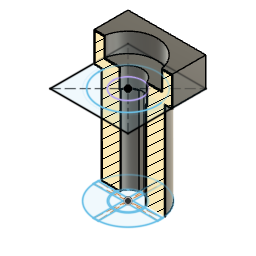
Expansion Anchor v8 (Autodesk Fusion 360 design; units mm, degrees)
Autodesk Fusion 360 part; units mm, degrees
note: some values were not read from the file. Set by a fixed rule: which sketch regions a step uses.
sketch "Schizzo1" plane through (0, 0, 0) normal (0, 0, 1) x (1, 0, 0)
  circle A0 centre (10.2944, 3.2873) radius 1.4
  circle A1 centre (10.2944, 3.2873) radius 3.3
  line L0 (13.5944, 3.0373) -> (6.9944, 3.0373)
  line L1 (6.9944, 3.0373) -> (6.9944, 3.5373)
  line L2 (6.9944, 3.5373) -> (13.5944, 3.5373)
  line L3 (13.5944, 3.5373) -> (13.5944, 3.0373)
  line L4 (13.5944, 3.0373) -> (6.9944, 3.5373) construction
  line L5 (6.9944, 3.0373) -> (13.5944, 3.5373) construction
  line L6 (10.5444, -0.0127) -> (10.0444, -0.0127)
  line L7 (10.0444, -0.0127) -> (10.0444, 6.5873)
  line L8 (10.0444, 6.5873) -> (10.5444, 6.5873)
  line L9 (10.5444, 6.5873) -> (10.5444, -0.0127)
  line L10 (10.5444, -0.0127) -> (10.0444, 6.5873) construction
  line L11 (10.0444, -0.0127) -> (10.5444, 6.5873) construction
  circle A2 centre (10.2944, 3.2873) radius 1.5
  point P0 (10.2944, 3.2873)
  point P1 (10.2944, 3.2873)
  dimension "d1" = 2.8
  dimension "d2" = 6.6
  dimension "d3" = 0.5
  dimension "d4" = 0.5
  dimension "d16" = 3
  constraint concentric A0 A1
  constraint horizontal L0
  constraint perpendicular L0 L1
  constraint parallel L0 L2
  constraint parallel L1 L3
  constraint coincident L4 P1
  constraint coincident L5 P1
  constraint coincident P0 A0.centre
  constraint horizontal L6
  constraint perpendicular L6 L7
  constraint parallel L6 L8
  constraint parallel L7 L9
  constraint coincident L10 P1
  constraint coincident L11 P1
  constraint coincident P1 P0
  constraint tangent A1 L1
  constraint tangent A1 L8
  constraint concentric A1 A2
  measures "d1" diameter of A0
  measures "d2" diameter of A1
  measures "d3" distance of L0.end L1.end
  measures "d4" distance of L7.end L8.end
  measures "d16" diameter of A2
extrude "Estrusione1" add sketch "Schizzo1" along normal blind 9 contours A0 L2 L9 A2 | A0 L0 L9 A2 | A1 L2 L9 A2 | A1 L0 L9 A2 | A0 L2 L7 A2 | A0 L0 L7 A2 | A1 L2 L7 A2 | A1 L0 L7 A2 makes body 1 at (7.1541, 4.3014, 6) makes body 2 at (7.5637, 1.4344, 6) makes body 3 at (12.397, 5.8308, 6) makes body 4 at (13.3249, 1.9811, 6)
extrude "Estrusione2" add sketch "Schizzo1" along normal blind 1 from surface at 9 contours A1 L2 L9 A2 | A1 L0 L2 A2 | A1 L0 L9 A2 | A1 L7 L9 A2 | A1 L7 L9 A2 | A1 L2 L7 A2 | A1 L0 L7 A2 | A1 L0 L2 A2 bodies 1 2 3 4
sketch "Schizzo2" plane through (0, 0, 10) normal (0, 0, 1) x (-1, 0, 0)
  circle A0 centre (-10.2944, -3.2873) radius 3.3
  line L0 (-14.2944, 0.7127) -> (-6.2944, 0.7127)
  line L1 (-6.2944, 0.7127) -> (-6.2944, -7.2873)
  line L2 (-6.2944, -7.2873) -> (-14.2944, -7.2873)
  line L3 (-14.2944, -7.2873) -> (-14.2944, 0.7127)
  line L4 (-14.2944, 0.7127) -> (-6.2944, -7.2873) construction
  line L5 (-6.2944, 0.7127) -> (-14.2944, -7.2873) construction
  circle A1 centre (-10.2944, -3.2873) radius 3
  circle A2 centre (-10.2944, -3.2873) radius 1.5
  point P0 (-10.2944, -3.2873)
  dimension "d10" = 8
  dimension "d11" = 8
  dimension "d13" = 6
  constraint horizontal L0
  constraint perpendicular L0 L1
  constraint parallel L0 L2
  constraint parallel L1 L3
  constraint coincident L4 P0
  constraint coincident L5 P0
  constraint coincident P0 A0.centre
  measures "d10" distance of L1.end L2.end
  measures "d11" distance of L0.end L1.end
  measures "d13" diameter of A1
extrude "Estrusione3" add sketch "Schizzo2" along normal blind 3 contours A0 | L0 L1 L2 L3 bodies 1
extrude "Estrusione4" add sketch "Schizzo2" along normal blind 1 contours A1 bodies 1
